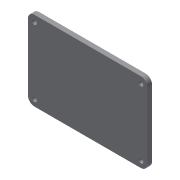
# Autodesk Inventor part: cellSTORM_v5_miniElectronics_lid
Saved by Autodesk Inventor 2019.4 (Build 234330000, 330)
## iProperties
Created: 2020-06-15
Part Number: cellSTORM_v5_miniElectronics_lid
Material: Generic
Document SubType Name: Modeling
Designer: diederichbenedict
Density: 1 g/cm^3
Appearance: White
Author: diederichbenedict
Autodesk Inventor part; units mm, degrees
ref_plane "YZ Plane" through (0, 0, 0) normal (1, 0, 0) x (0, 1, 0)
ref_plane "XZ Plane" through (0, 0, 0) normal (0, 1, 0) x (-1, 0, 0)
ref_plane "XY Plane" through (0, 0, 0) normal (0, 0, 1) x (1, 0, 0)
sketch "Sketch1" plane through (0, 0, 0) normal (0, 0, 1) x (1, 0, 0)
  circle A0 centre (67, 0) radius 1.5 projected
  circle A1 centre (67, 0) radius 4 projected
  circle A2 centre (67, -42) radius 1.5 projected
  circle A3 centre (67, -42) radius 4 projected
  circle A4 centre (0, -42) radius 1.5 projected
  circle A5 centre (0, -42) radius 4 projected
  circle A6 centre (0, 0) radius 1.5 projected
  circle A7 centre (0, 0) radius 4 projected
  line L0 (67, 4) -> (0, 4)
  line L1 (-4, 0) -> (-4, -42)
  line L2 (0, -46) -> (67, -46)
  line L3 (71, -42) -> (71, 0)
  point P0 (0, 0)
  constraints: 8 end point, 8 point on circle, 3 tangent, 1 perpendicular
extrude "Extrusion1" add sketch "Sketch1" along normal blind 3 contours A0 | A1 | L3 A3 L2 A5 L1 A7 L0 A1 | A3 | A7 | A5 | A2 | A4 | A6
sketch "Sketch2" plane through (0, 0, 3) normal (0, 0, 1) x (1, 0, 0)
  line L0 (67, 4) -> (0, 4) projected
  arc A0 (0, 4) -> (-4, 0) centre (0, 0) ccw projected
  line L1 (-4, 0) -> (-4, -42) projected
  arc A1 (-4, -42) -> (0, -46) centre (0, -42) ccw projected
  line L2 (0, -46) -> (67, -46) projected
  arc A2 (67, -46) -> (71, -42) centre (67, -42) ccw projected
  line L3 (71, -42) -> (71, 0) projected
  arc A3 (71, 0) -> (67, 4) centre (67, 0) ccw projected
  circle A4 centre (67, 0) radius 1.5 projected
  circle A5 centre (67, -42) radius 1.5 projected
  circle A6 centre (0, -42) radius 1.5 projected
  circle A7 centre (0, 0) radius 1.5 projected
  point P0 (0, 0)
extrude "Extrusion2" cut sketch "Sketch2" against normal through all contours A4 | A5 | A6 | A7
body "Solid1"
